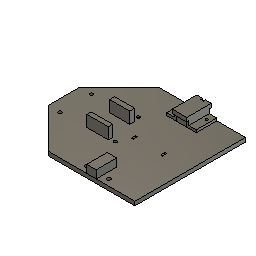
Chassis_v1 v17 (Autodesk Fusion 360 design; units mm, degrees)
Autodesk Fusion 360 part; units mm, degrees
sketch "Sketch1" plane through (0, 0, 0) normal (0, 1, 0) x (1, 0, 0) in component "Chassis"
  line L0 (0, 0) -> (160, 0)
  line L1 (160, 0) -> (160, -140)
  line L2 (160, -140) -> (0, -140)
  line L3 (0, -140) -> (0, 0)
  dimension "d1" = 160
  dimension "d2" = 140
  constraint horizontal L0
  constraint vertical L1
  constraint horizontal L2
  constraint vertical L3
  constraint coincident L0.start L3.end
  measures "d1" distance of L0.start L0.end
  measures "d2" distance of L0.start L2.end
extrude "Extrude1" add sketch "Sketch1" along normal blind 5.08 makes body 1 in component "Chassis"
sketch "Sketch2" plane through (0, 5.08, 0) normal (0, 1, 0) x (-1, 0, 0) in component "Chassis"
  line L0 (0, 140) -> (-160, 140)
  line L1 (-160, 140) -> (-160, 0)
  line L2 (-160, 0) -> (0, 0)
  line L3 (0, 0) -> (0, 140)
  line L4 (-80, 0) -> (-80, 140) construction
  line L5 (0, 70) -> (-160, 70) construction
  line L6 (-160, 0) -> (0, 140) construction
  line L7 (0, 0) -> (-160, 140) construction
  circle A0 centre (-15, 50.275) radius 2
  circle A1 centre (-15, 89.725) radius 2
  line L8 (-15, 50.275) -> (-15, 89.725) construction
  line L9 (-15, 70) -> (-20, 70) construction
  dimension "d5" = 4
  dimension "d6" = 4
  dimension "d7" = 39.45
  dimension "d8" = 15
  dimension "d9" = 15
  constraint midpoint L2 L4.start
  constraint midpoint L0 L4.end
  constraint midpoint L3 L5.start
  constraint midpoint L1 L5.end
  constraint coincident L1.end L2.start
  constraint coincident L0.start L3.end
  constraint coincident L2.end L3.start
  constraint coincident L0.end L1.start
  constraint coincident A0.centre L8.start
  constraint coincident A1.centre L8.end
  constraint midpoint L8 L9.start
  constraint perpendicular L8 L9
  constraint collinear L5 L9
  measures "d5" diameter of A0
  measures "d6" diameter of A1
  measures "d7" vertical distance of A0.centre A1.centre
  measures "d8" distance of L3 A0.centre
  measures "d9" distance of L3 A1.centre
extrude "Extrude2" cut sketch "Sketch2" against normal blind 5.08 contours A0 | A1 bodies 1 in component "Chassis"
sketch "Sketch3" plane through (0, 5.08, 0) normal (0, 1, 0) x (-1, 0, 0) in component "Chassis"
  circle A0 centre (-15, 50.275) radius 2
  circle A1 centre (-15, 89.725) radius 2
  line L0 (0, 140) -> (-160, 140)
  line L1 (-160, 140) -> (-160, 0)
  line L2 (-160, 0) -> (0, 0)
  line L3 (0, 0) -> (0, 140)
  line L4 (-30, 71.55) -> (-84, 71.55) construction
  line L5 (-84, 71.55) -> (-84, 109.55) construction
  line L6 (-84, 109.55) -> (-30, 109.55) construction
  line L7 (-30, 109.55) -> (-30, 71.55) construction
  circle A2 centre (-82.2, 86.84) radius 2
  circle A3 centre (-42.6, 80.03) radius 2
  line L8 (0, 70) -> (-160, 70) construction
  dimension "d12" = 54
  dimension "d13" = 38
  dimension "d14" = 4
  dimension "d15" = 22.71
  dimension "d16" = 1.8
  dimension "d17" = 4
  dimension "d18" = 8.48
  dimension "d19" = 12.6
  dimension "d20" = 30.45
  dimension "d21" = 30
  constraint horizontal L4
  constraint vertical L5
  constraint horizontal L6
  constraint vertical L7
  constraint midpoint L3 L8.start
  constraint midpoint L1 L8.end
  measures "d12" distance of L5.end L6.end
  measures "d13" distance of L4.start L6.end
  measures "d14" diameter of A2
  measures "d15" distance of L6 A2.centre
  measures "d16" distance of L5 A2.centre
  measures "d17" diameter of A3
  measures "d18" distance of L4 A3.centre
  measures "d19" distance of L7 A3.centre
  measures "d20" distance of L0 L6
  measures "d21" distance of L3 L7
extrude "Extrude3" cut sketch "Sketch3" against normal blind 5.08 contours A2 | A3 bodies 1 in component "Chassis"
sketch "Sketch4" plane through (0, 0, 0) normal (0, -1, 0) x (1, 0, 0) in component "Chassis"
  circle A0 centre (42.6, 80.03) radius 2
  circle A1 centre (82.2, 86.84) radius 2
  circle A2 centre (15, 50.275) radius 2
  circle A3 centre (15, 89.725) radius 2
  line L0 (160, 140) -> (0, 140)
  line L1 (0, 140) -> (0, 0)
  line L2 (0, 0) -> (160, 0)
  line L3 (160, 0) -> (160, 140)
  circle A4 centre (42.6, 80.03) radius 5
  circle A5 centre (82.2, 86.84) radius 5
  point P0 (42.6, 80.03)
  point P1 (82.2, 86.84)
  dimension "d105" = 10
  dimension "d106" = 10
  constraint coincident P0 A0.centre
  constraint coincident P1 A1.centre
  constraint concentric A1 A5
  measures "d105" diameter of A4
  measures "d106" diameter of A5
extrude "Extrude10" cut sketch "Sketch4" against normal blind 3 contours A4 | A5 bodies 1 in component "Chassis"
extrude "Extrude4" cut sketch "Sketch4" against normal blind 3 contours A0 | A4 | A5 bodies 1 in component "Chassis"
chamfer "Chamfer1" distance 50 angle 45 2 edges at (0, 2.54, 140) (0, 2.54, 0) on bodies 1 in component "Chassis"
sketch "Sketch5" plane through (0, 5.08, 0) normal (0, 1, 0) x (-1, 0, 0) in component "Chassis"
  line L0 (-93, 41.4) -> (-123, 41.4) construction
  line L1 (-123, 41.4) -> (-123, 98.6) construction
  line L2 (-123, 98.6) -> (-93, 98.6) construction
  line L3 (-93, 98.6) -> (-93, 41.4) construction
  line L4 (-123, 70) -> (-93, 70) construction
  line L5 (0, 70) -> (-160, 70) construction
  line L6 (-84, 71.55) -> (-84, 109.55)
  line L7 (-91, 72.5) -> (-88.5, 72.5)
  line L8 (-88.5, 72.5) -> (-88.5, 67.5)
  line L9 (-88.5, 67.5) -> (-91, 67.5)
  line L10 (-91, 67.5) -> (-91, 72.5)
  line L11 (-91, 72.5) -> (-88.5, 67.5) construction
  line L12 (-88.5, 72.5) -> (-91, 67.5) construction
  line L13 (-128, 72.5) -> (-125.5, 72.5)
  line L14 (-125.5, 72.5) -> (-125.5, 67.5)
  line L15 (-125.5, 67.5) -> (-128, 67.5)
  line L16 (-128, 67.5) -> (-128, 72.5)
  line L17 (-128, 72.5) -> (-125.5, 67.5) construction
  line L18 (-125.5, 72.5) -> (-128, 67.5) construction
  point P0 (-89.75, 70)
  point P1 (-126.75, 70)
  dimension "d29" = 30
  dimension "d30" = 57.2
  dimension "d31" = 9
  dimension "d32" = 2.5
  dimension "d33" = 5
  dimension "d34" = 2
  dimension "d35" = 2.5
  dimension "d36" = 5
  dimension "d37" = 2.5
  constraint horizontal L0
  constraint vertical L1
  constraint horizontal L2
  constraint vertical L3
  constraint midpoint L1 L4.start
  constraint midpoint L3 L4.end
  constraint collinear L4 L5
  constraint horizontal L7
  constraint perpendicular L7 L8
  constraint parallel L7 L9
  constraint parallel L8 L10
  constraint coincident L11 P0
  constraint coincident L12 P0
  constraint coincident L5 P0
  constraint horizontal L13
  constraint perpendicular L13 L14
  constraint parallel L13 L15
  constraint parallel L14 L16
  constraint coincident L17 P1
  constraint coincident L18 P1
  constraint coincident L5 P1
  measures "d29" distance of L0.start L0.end
  measures "d30" distance of L0.start L2.end
  measures "d31" distance of L3 L6
  measures "d32" distance of L8.end L9.end
  measures "d33" distance of L7.end L8.end
  measures "d34" distance of L3 L10
  measures "d35" distance of L14.end L15.end
  measures "d36" distance of L13.end L14.end
  measures "d37" distance of L1 L14
extrude "Extrude5" cut sketch "Sketch5" against normal blind 5.08 bodies 1 in component "Chassis"
sketch "Sketch6" plane through (0, 5.08, 0) normal (0, 1, 0) x (-1, 0, 0) in component "Chassis"
  line L0 (-47, 43.05) -> (-72.4, 43.05) construction
  line L1 (-72.4, 43.05) -> (-72.4, 68.45) construction
  line L2 (-72.4, 68.45) -> (-47, 68.45) construction
  line L3 (-47, 68.45) -> (-47, 43.05) construction
  line L4 (0, 70) -> (-160, 70)
  line L5 (0, 0) -> (0, 140)
  circle A0 centre (-49.54, 45.59) radius 2
  circle A1 centre (-69.86, 45.59) radius 2
  line L6 (-59.7, 43.05) -> (-59.7, 68.45) construction
  line L7 (-47, 55.75) -> (-72.4, 55.75) construction
  line L8 (-72.4, 58.925) -> (-47, 58.925)
  line L9 (-47, 58.925) -> (-47, 52.575)
  line L10 (-47, 52.575) -> (-72.4, 52.575)
  line L11 (-72.4, 52.575) -> (-72.4, 58.925)
  line L12 (-72.4, 58.925) -> (-47, 52.575) construction
  line L13 (-47, 58.925) -> (-72.4, 52.575) construction
  point P0 (-59.7, 55.75)
  dimension "d40" = 25.4
  dimension "d41" = 25.4
  dimension "d42" = 1.55
  dimension "d43" = 47
  dimension "d44" = 4
  dimension "d45" = 2.54
  dimension "d46" = 2.54
  dimension "d47" = 4
  dimension "d48" = 2.54
  dimension "d49" = 2.54
  dimension "d52" = 6.35
  constraint horizontal L0
  constraint vertical L1
  constraint horizontal L2
  constraint vertical L3
  constraint midpoint L0 L6.start
  constraint midpoint L2 L6.end
  constraint midpoint L3 L7.start
  constraint midpoint L1 L7.end
  constraint horizontal L8
  constraint perpendicular L8 L9
  constraint parallel L8 L10
  constraint parallel L9 L11
  constraint coincident L12 P0
  constraint coincident L13 P0
  constraint midpoint L7 P0
  measures "d40" distance of L0.start L0.end
  measures "d41" distance of L0.start L2.end
  measures "d42" distance of L2 L4
  measures "d43" distance of L3 L5
  measures "d44" diameter of A0
  measures "d45" distance of L0 A0.centre
  measures "d46" distance of L3 A0.centre
  measures "d47" diameter of A1
  measures "d48" distance of L0 A1.centre
  measures "d49" distance of L1 A1.centre
  measures "d52" distance of L8.end L9.end
extrude "Extrude7" add sketch "Sketch6" along normal blind 14.45 contours L8 L9 L10 L11 bodies 1 in component "Chassis"
extrude "Extrude6" cut sketch "Sketch6" against normal blind 5.08 contours A0 | A1 bodies 1 in component "Chassis"
sketch "Sketch7" plane through (0, 0, 0) normal (0, -1, 0) x (1, 0, 0) in component "Chassis"
  circle A0 centre (49.54, 45.59) radius 2
  circle A1 centre (69.86, 45.59) radius 2
  line L0 (88.5, 67.5) -> (88.5, 72.5)
  line L1 (88.5, 72.5) -> (91, 72.5)
  line L2 (91, 72.5) -> (91, 67.5)
  line L3 (91, 67.5) -> (88.5, 67.5)
  line L4 (125.5, 67.5) -> (125.5, 72.5)
  line L5 (125.5, 72.5) -> (128, 72.5)
  line L6 (128, 72.5) -> (128, 67.5)
  line L7 (128, 67.5) -> (125.5, 67.5)
  line L8 (0, 50) -> (50, 0)
  line L9 (50, 0) -> (160, 0)
  line L10 (160, 0) -> (160, 140)
  line L11 (160, 140) -> (50, 140)
  line L12 (50, 140) -> (0, 90)
  line L13 (0, 90) -> (0, 50)
  circle A2 centre (15, 50.275) radius 2
  circle A3 centre (15, 89.725) radius 2
  circle A4 centre (42.6, 80.03) radius 5
  circle A5 centre (82.2, 86.84) radius 5
  circle A6 centre (49.54, 45.59) radius 5
  circle A7 centre (69.86, 45.59) radius 5
  point P0 (49.54, 45.59)
  point P1 (69.86, 45.59)
  dimension "d109" = 10
  dimension "d110" = 10
  constraint coincident P0 A0.centre
  constraint coincident P1 A1.centre
  constraint concentric A0 A6
  measures "d109" diameter of A6
  measures "d110" diameter of A7
extrude "Extrude11" cut sketch "Sketch7" against normal blind 3 contours A6 | A7 bodies 1 in component "Chassis"
extrude "Extrude8" cut sketch "Sketch7" against normal blind 3 contours A0 | A6 | A7 bodies 1 in component "Chassis"
sketch "Sketch1 (2)" plane through (0, 5.08, 0) normal (0, 1, 0) x (-1, 0, 0) in component "Motor_Right"
  circle A0 centre (-49.54, 45.59) radius 2
  circle A1 centre (-69.86, 45.59) radius 2
  line L0 (-72.4, 52.575) -> (-72.4, 58.925)
  line L1 (-72.4, 58.925) -> (-47, 58.925)
  line L2 (-47, 58.925) -> (-47, 52.575)
  line L3 (-47, 52.575) -> (-72.4, 52.575)
  line L4 (-88.5, 72.5) -> (-88.5, 67.5)
  line L5 (-88.5, 67.5) -> (-91, 67.5)
  line L6 (-91, 67.5) -> (-91, 72.5)
  line L7 (-91, 72.5) -> (-88.5, 72.5)
  line L8 (-125.5, 72.5) -> (-125.5, 67.5)
  line L9 (-125.5, 67.5) -> (-128, 67.5)
  line L10 (-128, 67.5) -> (-128, 72.5)
  line L11 (-128, 72.5) -> (-125.5, 72.5)
  circle A2 centre (-42.6, 80.03) radius 2
  circle A3 centre (-82.2, 86.84) radius 2
  circle A4 centre (-15, 50.275) radius 2
  circle A5 centre (-15, 89.725) radius 2
  line L12 (-50, 0) -> (0, 50)
  line L13 (0, 50) -> (0, 90)
  line L14 (0, 90) -> (-50, 140)
  line L15 (-50, 140) -> (-160, 140)
  line L16 (-160, 140) -> (-160, 0)
  line L17 (-160, 0) -> (-50, 0)
  line L18 (-105, 140) -> (-105, 70) construction
  line L19 (-105, 140) -> (-99, 140) construction
  line L20 (-99, 140) -> (-111, 140)
  line L21 (-111, 140) -> (-111, 114)
  line L22 (-111, 114) -> (-99, 114)
  line L23 (-99, 114) -> (-99, 140)
  dimension "d59" = 26
  dimension "d60" = 12
  dimension "d61" = 49
  constraint midpoint L15 L18.start
  constraint perpendicular L9 L18
  constraint coincident L15 L19.end
  constraint perpendicular L18 L19
  constraint horizontal L20
  constraint vertical L21
  constraint horizontal L22
  constraint vertical L23
  measures "d59" distance of L19.end L22.end
  measures "d60" distance of L19.end L20.end
  measures "d61" distance of L16 L21
extrude "Extrude1'" add sketch "Sketch1 (2)" along normal blind 10 separate body contours L15 L20 L21 L22 L23 makes body 2 in component "Motor_Right"
sketch "Sketch1 (3)" plane through (0, 5.08, 0) normal (0, 1, 0) x (-1, 0, 0) in component "Motor_Left"
  circle A0 centre (-49.54, 45.59) radius 2
  circle A1 centre (-69.86, 45.59) radius 2
  line L0 (-72.4, 52.575) -> (-72.4, 58.925)
  line L1 (-72.4, 58.925) -> (-47, 58.925)
  line L2 (-47, 58.925) -> (-47, 52.575)
  line L3 (-47, 52.575) -> (-72.4, 52.575)
  line L4 (-88.5, 72.5) -> (-88.5, 67.5)
  line L5 (-88.5, 67.5) -> (-91, 67.5)
  line L6 (-91, 67.5) -> (-91, 72.5)
  line L7 (-91, 72.5) -> (-88.5, 72.5)
  line L8 (-125.5, 72.5) -> (-125.5, 67.5)
  line L9 (-125.5, 67.5) -> (-128, 67.5)
  line L10 (-128, 67.5) -> (-128, 72.5)
  line L11 (-128, 72.5) -> (-125.5, 72.5)
  circle A2 centre (-42.6, 80.03) radius 2
  circle A3 centre (-82.2, 86.84) radius 2
  circle A4 centre (-15, 50.275) radius 2
  circle A5 centre (-15, 89.725) radius 2
  line L12 (-50, 0) -> (0, 50)
  line L13 (0, 50) -> (0, 90)
  line L14 (0, 90) -> (-50, 140)
  line L15 (-50, 140) -> (-160, 140)
  line L16 (-160, 140) -> (-160, 0)
  line L17 (-160, 0) -> (-50, 0)
  line L18 (-105, 0) -> (-105, 70) construction
  line L19 (-105, 0) -> (-99, 0) construction
  line L20 (-99, 0) -> (-111, 0)
  line L21 (-111, 0) -> (-111, 26)
  line L22 (-111, 26) -> (-99, 26)
  line L23 (-99, 26) -> (-99, 0)
  dimension "d64" = 6
  dimension "d65" = 12
  dimension "d66" = 26
  constraint midpoint L17 L18.start
  constraint perpendicular L17 L18
  constraint perpendicular L18 L19
  constraint horizontal L20
  constraint vertical L21
  constraint horizontal L22
  constraint vertical L23
  measures "d64" distance of L18.start L19.end
  measures "d65" distance of L19.end L20.end
  measures "d66" distance of L19.end L22.end
extrude "Extrude1''" add sketch "Sketch1 (3)" along normal blind 10 separate body contours L17 L20 L21 L22 L23 makes body 3 in component "Motor_Left"
sketch "Sketch1 (4)" plane through (0, 0, 0) normal (0, 0, -1) x (-1, 0, 0) in component "Motor_Bracket_Left"
  line L0 (-111, 5.08) -> (-99, 5.08)
  line L1 (-99, 5.08) -> (-99, 15.08)
  line L2 (-99, 15.08) -> (-111, 15.08)
  line L3 (-111, 15.08) -> (-111, 5.08)
  line L4 (-111.03, 15.11) -> (-111.03, 5.08)
  line L5 (-160, 5.08) -> (-50, 5.08)
  line L6 (-111.03, 5.08) -> (-123.73, 5.08)
  line L7 (-123.73, 5.08) -> (-123.73, 8.255)
  line L8 (-123.73, 8.255) -> (-114.205, 8.255)
  line L9 (-114.205, 8.255) -> (-114.205, 18.285)
  line L10 (-105, 18.285) -> (-114.205, 18.285)
  line L11 (-105, 15.11) -> (-111.03, 15.11)
  line L12 (-105, 18.285) -> (-95.795, 18.285)
  line L13 (-95.795, 8.255) -> (-95.795, 18.285)
  line L14 (-86.27, 8.255) -> (-95.795, 8.255)
  line L15 (-86.27, 5.08) -> (-86.27, 8.255)
  line L16 (-105, 15.11) -> (-98.97, 15.11)
  line L17 (-98.97, 15.11) -> (-98.97, 5.08)
  line L18 (-98.97, 5.08) -> (-86.27, 5.08)
  dimension "d70" = 12.7
  dimension "d71" = 3.175
  dimension "d72" = 9.525
  dimension "d73" = 10.03
  dimension "d74" = 10.03
  dimension "d75" = 18.41
  dimension "d76" = 37.46
  dimension "d77" = 13.205
  constraint parallel L3 L4
  constraint coincident L4.end L5
  constraint perpendicular L4 L6
  constraint perpendicular L5 L7
  constraint perpendicular L7 L8
  constraint perpendicular L8 L9
  constraint perpendicular L9 L10
  measures "d70" distance of L4.end L6.end
  measures "d71" distance of L6.end L7.end
  measures "d72" distance of L7.end L8.end
  measures "d73" distance of L4.end L4.start
  measures "d74" distance of L8.end L9.end
  measures "d75" distance of L9 L13
  measures "d76" distance of L7 L15
  measures "d77" distance of L12 L18
extrude "Extrude1'''" add sketch "Sketch1 (4)" against normal blind 16 separate body contours L4 L5 L6 L7 L8 L9 L10 L11 L12 L13 L14 L15 L16 L17 L18 makes body 4 in component "Motor_Bracket_Left"
sketch "Sketch2 (2)" plane through (0, 0, 0) normal (0, 0, -1) x (-1, 0, 0) in component "Motor_Bracket_Left"
  line L0 (-111.03, 15.11) -> (-98.97, 15.11)
  line L1 (-98.97, 15.11) -> (-98.97, 5.08)
  line L2 (-98.97, 5.08) -> (-86.27, 5.08)
  line L3 (-86.27, 5.08) -> (-86.27, 8.255)
  line L4 (-86.27, 8.255) -> (-95.795, 8.255)
  line L5 (-95.795, 8.255) -> (-95.795, 18.285)
  line L6 (-95.795, 18.285) -> (-114.205, 18.285)
  line L7 (-114.205, 18.285) -> (-114.205, 8.255)
  line L8 (-114.205, 8.255) -> (-123.73, 8.255)
  line L9 (-123.73, 8.255) -> (-123.73, 5.08)
  line L10 (-123.73, 5.08) -> (-111.03, 5.08)
  line L11 (-111.03, 5.08) -> (-111.03, 15.11)
  line L12 (-114.205, 18.285) -> (-95.795, 18.285)
  line L13 (-95.795, 18.285) -> (-95.795, 13.27)
  line L14 (-95.795, 13.27) -> (-114.205, 13.27)
  line L15 (-114.205, 13.27) -> (-114.205, 18.285)
  dimension "d121" = 5.015
  dimension "d122" = 18.41
  constraint horizontal L12
  constraint vertical L13
  constraint horizontal L14
  constraint vertical L15
  constraint midpoint L5 L13.end
  constraint coincident L6.end L7.start
  measures "d121" distance of L6.end L14.end
  measures "d122" distance of L6.end L5.end
extrude "Extrude2'" add sketch "Sketch2 (2)" along normal blind 2.5 contours L0 L1 L5 L6 L7 L11 L12 L13 L14 L15 | L0 L1 L11 L14 bodies 4 in component "Motor_Bracket_Left"
sketch "Sketch3 (2)" plane through (0, 13.27, 0) normal (0, -1, 0) x (1, 0, 0) in component "Motor_Bracket_Left"
  line L0 (98.97, 0) -> (95.795, 0)
  line L1 (95.795, 0) -> (95.795, -2.5)
  line L2 (95.795, -2.5) -> (114.205, -2.5)
  line L3 (114.205, -2.5) -> (114.205, 0)
  line L4 (114.205, 0) -> (111.03, 0)
  line L5 (111.03, 0) -> (98.97, 0)
  line L6 (105, -2.5) -> (105, 0) construction
  line L7 (95.795, -1.25) -> (114.205, -1.25) construction
  line L8 (109.875, -2.5) -> (100.125, -2.5)
  line L9 (100.125, -2.5) -> (100.125, 0)
  line L10 (100.125, 0) -> (109.875, 0)
  line L11 (109.875, 0) -> (109.875, -2.5)
  line L12 (109.875, -2.5) -> (100.125, 0) construction
  line L13 (100.125, -2.5) -> (109.875, 0) construction
  point P0 (105, -1.25)
  dimension "d82" = 9.75
  constraint midpoint L2 L6.start
  constraint midpoint L5 L6.end
  constraint midpoint L1 L7.start
  constraint midpoint L3 L7.end
  constraint horizontal L8
  constraint perpendicular L8 L9
  constraint parallel L8 L10
  constraint parallel L9 L11
  constraint coincident L12 P0
  constraint coincident L13 P0
  constraint midpoint L7 P0
  measures "d82" distance of L9.end L10.end
extrude "Extrude3'" cut sketch "Sketch3 (2)" against normal blind 1.84 contours L2 L5 L8 L9 L10 L11 bodies 4 in component "Motor_Bracket_Left"
sketch "Sketch4 (2)" plane through (0, 8.255, 0) normal (0, 1, 0) x (-1, 0, 0) in component "Motor_Bracket_Left"
  line L0 (-123.73, 0) -> (-114.205, 0)
  line L1 (-114.205, 0) -> (-114.205, 16)
  line L2 (-114.205, 16) -> (-123.73, 16)
  line L3 (-123.73, 16) -> (-123.73, 0)
  line L4 (-114.205, 0) -> (-123.73, 16) construction
  line L5 (-123.73, 0) -> (-114.205, 16) construction
  circle A0 centre (-118.9675, 8) radius 1.5
  dimension "d85" = 3
  constraint coincident L0.end L1.start
  constraint coincident L2.end L3.start
  constraint coincident L0.start L3.end
  constraint coincident L1.end L2.start
  constraint midpoint L5 A0.centre
  measures "d85" diameter of A0
extrude "Extrude4'" cut sketch "Sketch4 (2)" against normal blind 3.175 contours A0 bodies 4 in component "Motor_Bracket_Left"
sketch "Sketch5 (2)" plane through (0, 8.255, 0) normal (0, 1, 0) x (-1, 0, 0) in component "Motor_Bracket_Left"
  line L0 (-95.795, 0) -> (-86.27, 0)
  line L1 (-86.27, 0) -> (-86.27, 16)
  line L2 (-86.27, 16) -> (-95.795, 16)
  line L3 (-95.795, 16) -> (-95.795, 0)
  line L4 (-86.27, 16) -> (-95.795, 0) construction
  line L5 (-86.27, 0) -> (-95.795, 16) construction
  circle A0 centre (-91.0325, 8) radius 1.5
  dimension "d88" = 3
  constraint coincident L1.end L2.start
  constraint coincident L0.start L3.end
  constraint coincident L0.end L1.start
  constraint coincident L2.end L3.start
  constraint midpoint L4 A0.centre
  measures "d88" diameter of A0
extrude "Extrude5'" cut sketch "Sketch5 (2)" against normal blind 3.175 contours A0 bodies 4 in component "Motor_Bracket_Left"
extrude "Extrude6'" add 1 faces at (107.01, 17.2267, 16) along direction (0, 0, 1) blind 10.03 on bodies 4 bodies 4 in component "Motor_Bracket_Left"
sketch "Sketch6 (2)" plane through (0, 0, 26.03) normal (0, 0, 1) x (1, 0, 0) in component "Motor_Bracket_Left"
  line L0 (98.97, 15.11) -> (111.03, 15.11)
  line L1 (111.03, 15.11) -> (111.03, 5.08)
  line L2 (111.03, 5.08) -> (123.73, 5.08)
  line L3 (123.73, 5.08) -> (123.73, 8.255)
  line L4 (123.73, 8.255) -> (114.205, 8.255)
  line L5 (114.205, 8.255) -> (114.205, 18.285)
  line L6 (114.205, 18.285) -> (95.795, 18.285)
  line L7 (95.795, 18.285) -> (95.795, 8.255)
  line L8 (95.795, 8.255) -> (86.27, 8.255)
  line L9 (86.27, 8.255) -> (86.27, 5.08)
  line L10 (86.27, 5.08) -> (98.97, 5.08)
  line L11 (98.97, 5.08) -> (98.97, 15.11)
  line L12 (95.795, 18.285) -> (114.205, 18.285)
  line L13 (114.205, 18.285) -> (114.205, 13.27)
  line L14 (114.205, 13.27) -> (95.795, 13.27)
  line L15 (95.795, 13.27) -> (95.795, 18.285)
  dimension "d123" = 18.41
  dimension "d124" = 5.015
  constraint horizontal L12
  constraint vertical L13
  constraint horizontal L14
  constraint vertical L15
  constraint midpoint L5 L13.end
  constraint coincident L6.end L7.start
  measures "d123" distance of L6.end L5.end
  measures "d124" distance of L5.end L13.end
extrude "Extrude7'" add sketch "Sketch6 (2)" along normal blind 2.5 contours L0 L1 L5 L6 L7 L11 L12 L13 L14 L15 | L0 L1 L11 L14 bodies 4 in component "Motor_Bracket_Left"
extrude "Extrude8'" cut 2 faces at (99.74, 14.4967, 0) (110.645, 14.4967, 0) along direction (0, 0, -1) blind 0.03 on bodies 4 bodies 4 in component "Motor_Bracket_Left"
sketch "Sketch8" plane through (0, 0, 0) normal (0, -1, 0) x (1, 0, 0) in component "Chassis"
  line L0 (88.5, 67.5) -> (88.5, 72.5)
  line L1 (88.5, 72.5) -> (91, 72.5)
  line L2 (91, 72.5) -> (91, 67.5)
  line L3 (91, 67.5) -> (88.5, 67.5)
  line L4 (125.5, 67.5) -> (125.5, 72.5)
  line L5 (125.5, 72.5) -> (128, 72.5)
  line L6 (128, 72.5) -> (128, 67.5)
  line L7 (128, 67.5) -> (125.5, 67.5)
  line L8 (0, 50) -> (50, 0)
  line L9 (50, 0) -> (160, 0)
  line L10 (160, 0) -> (160, 140)
  line L11 (160, 140) -> (50, 140)
  line L12 (50, 140) -> (0, 90)
  line L13 (0, 90) -> (0, 50)
  circle A0 centre (15, 50.275) radius 2
  circle A1 centre (15, 89.725) radius 2
  circle A2 centre (118.9675, 8) radius 1.5 construction
  circle A3 centre (91.0325, 8) radius 1.5 construction
  circle A4 centre (118.9675, 8) radius 2.15
  circle A5 centre (91.0325, 8) radius 2.15
  line L14 (0, 70) -> (160, 70) construction
  circle A6 centre (118.9675, 132) radius 2.15
  circle A7 centre (91.0325, 132) radius 2.15
  circle A8 centre (91.0325, 132) radius 2.15
  circle A9 centre (118.9675, 132) radius 2.15
  circle A10 centre (91.0325, 8) radius 2.15
  circle A11 centre (118.9675, 8) radius 2.15
  circle A12 centre (42.6, 80.03) radius 5
  circle A13 centre (82.2, 86.84) radius 5
  circle A14 centre (69.86, 45.59) radius 5
  circle A15 centre (49.54, 45.59) radius 5
  dimension "d97" = 4.3
  dimension "d98" = 4.3
  constraint concentric A2 A4
  constraint concentric A3 A5
  constraint midpoint L13 L14.start
  constraint midpoint L10 L14.end
  constraint symmetric A4 L14 A6
  constraint symmetric A5 L14 A7
  constraint concentric A7 A8
  constraint concentric A6 A9
  constraint concentric A5 A10
  constraint concentric A2 A11
  measures "d97" diameter of A4
  measures "d98" diameter of A5
sketch "Sketch9" plane through (0, 5.08, 0) normal (0, 1, 0) x (-1, 0, 0) in component "Chassis"
  circle A0 centre (-49.54, 45.59) radius 2
  circle A1 centre (-69.86, 45.59) radius 2
  line L0 (-72.4, 52.575) -> (-72.4, 58.925)
  line L1 (-72.4, 58.925) -> (-47, 58.925)
  line L2 (-47, 58.925) -> (-47, 52.575)
  line L3 (-47, 52.575) -> (-72.4, 52.575)
  line L4 (-88.5, 72.5) -> (-88.5, 67.5)
  line L5 (-88.5, 67.5) -> (-91, 67.5)
  line L6 (-91, 67.5) -> (-91, 72.5)
  line L7 (-91, 72.5) -> (-88.5, 72.5)
  line L8 (-125.5, 72.5) -> (-125.5, 67.5)
  line L9 (-125.5, 67.5) -> (-128, 67.5)
  line L10 (-128, 67.5) -> (-128, 72.5)
  line L11 (-128, 72.5) -> (-125.5, 72.5)
  circle A2 centre (-42.6, 80.03) radius 2
  circle A3 centre (-82.2, 86.84) radius 2
  circle A4 centre (-15, 50.275) radius 2
  circle A5 centre (-15, 89.725) radius 2
  line L12 (-50, 0) -> (0, 50)
  line L13 (0, 50) -> (0, 90)
  line L14 (0, 90) -> (-50, 140)
  line L15 (-50, 140) -> (-160, 140)
  line L16 (-160, 140) -> (-160, 0)
  line L17 (-160, 0) -> (-50, 0)
  circle A6 centre (-91, 8) radius 2.15
  circle A7 centre (-119, 8) radius 2.15
  circle A8 centre (-91, 132) radius 2.15
  circle A9 centre (-119, 132) radius 2.15
  dimension "d99" = 4.3
  dimension "d100" = 4.3
  dimension "d101" = 4.3
  dimension "d102" = 4.3
  measures "d99" diameter of A6
  measures "d100" diameter of A7
  measures "d101" diameter of A8
  measures "d102" diameter of A9
extrude "Extrude9" cut sketch "Sketch9" against normal blind 3.43 contours A6 | A7 | A8 | A9 bodies 1 in component "Chassis"
sketch "Sketch7 (2)" plane through (0, 0, -2.5) normal (0, 0, -1) x (-1, 0, 0) in component "Motor_Bracket_Left"
  line L0 (-109.875, 13.27) -> (-109.875, 15.11)
  line L1 (-109.875, 15.11) -> (-100.125, 15.11)
  line L2 (-100.125, 15.11) -> (-100.125, 13.27)
  line L3 (-100.125, 13.27) -> (-95.795, 13.27)
  line L4 (-95.795, 13.27) -> (-95.795, 18.285)
  line L5 (-95.795, 18.285) -> (-114.205, 18.285)
  line L6 (-114.205, 18.285) -> (-114.205, 13.27)
  line L7 (-114.205, 13.27) -> (-109.875, 13.27)
  line L8 (-105, 15.11) -> (-105, 18.285) construction
  line L9 (-105, 16.6975) -> (-114.205, 16.6975) construction
  line L10 (-103.5, 15.11) -> (-106.5, 15.11)
  line L11 (-106.5, 15.11) -> (-106.5, 18.285)
  line L12 (-106.5, 18.285) -> (-103.5, 18.285)
  line L13 (-103.5, 18.285) -> (-103.5, 15.11)
  line L14 (-103.5, 15.11) -> (-106.5, 18.285) construction
  line L15 (-106.5, 15.11) -> (-103.5, 18.285) construction
  point P0 (-105, 16.6975)
  dimension "d113" = 3
  constraint midpoint L1 L8.start
  constraint midpoint L5 L8.end
  constraint midpoint L8 P0
  constraint coincident L6 L9.end
  constraint perpendicular L6 L9
  constraint horizontal L10
  constraint perpendicular L10 L11
  constraint parallel L10 L12
  constraint parallel L11 L13
  constraint coincident L14 P0
  constraint coincident L15 P0
  constraint coincident P0 L9.start
  measures "d113" distance of L11.end L12.end
extrude "Extrude9'" cut sketch "Sketch7 (2)" against normal blind 2.5 contours L1 L5 L10 L11 L12 L13 bodies 4 in component "Motor_Bracket_Left"
sketch "Sketch10" plane through (0, 5.08, 0) normal (0, 1, 0) x (-1, 0, 0) in component "Chassis"
  circle A0 centre (-119, 132) radius 2.15
  circle A1 centre (-91, 8) radius 2.15
  circle A2 centre (-91, 132) radius 2.15
  circle A3 centre (-119, 8) radius 2.15
  circle A4 centre (-49.54, 45.59) radius 2
  circle A5 centre (-69.86, 45.59) radius 2
  line L0 (-72.4, 52.575) -> (-72.4, 58.925)
  line L1 (-72.4, 58.925) -> (-47, 58.925)
  line L2 (-47, 58.925) -> (-47, 52.575)
  line L3 (-47, 52.575) -> (-72.4, 52.575)
  line L4 (-88.5, 72.5) -> (-88.5, 67.5)
  line L5 (-88.5, 67.5) -> (-91, 67.5)
  line L6 (-91, 67.5) -> (-91, 72.5)
  line L7 (-91, 72.5) -> (-88.5, 72.5)
  line L8 (-125.5, 72.5) -> (-125.5, 67.5)
  line L9 (-125.5, 67.5) -> (-128, 67.5)
  line L10 (-128, 67.5) -> (-128, 72.5)
  line L11 (-128, 72.5) -> (-125.5, 72.5)
  circle A6 centre (-42.6, 80.03) radius 2
  circle A7 centre (-82.2, 86.84) radius 2
  circle A8 centre (-15, 50.275) radius 2
  circle A9 centre (-15, 89.725) radius 2
  line L12 (-50, 0) -> (0, 50)
  line L13 (0, 50) -> (0, 90)
  line L14 (0, 90) -> (-50, 140)
  line L15 (-50, 140) -> (-160, 140)
  line L16 (-160, 140) -> (-160, 0)
  line L17 (-160, 0) -> (-50, 0)
  line L18 (-82.2, 86.84) -> (-42.6, 86.84) construction
  line L19 (-62.4, 86.84) -> (-62.4, 83) construction
  line L20 (-48.9, 84.09) -> (-75.9, 84.09)
  line L21 (-75.9, 84.09) -> (-75.9, 89.59)
  line L22 (-75.9, 89.59) -> (-48.9, 89.59)
  line L23 (-48.9, 89.59) -> (-48.9, 84.09)
  line L24 (-48.9, 84.09) -> (-75.9, 89.59) construction
  line L25 (-75.9, 84.09) -> (-48.9, 89.59) construction
  point P0 (-62.4, 86.84)
  dimension "d116" = 27
  dimension "d117" = 5.5
  dimension "d120" = 6.3
  constraint coincident A7.centre L18.start
  constraint horizontal L18
  constraint midpoint L18 P0
  constraint perpendicular L18 L19
  constraint horizontal L20
  constraint perpendicular L20 L21
  constraint parallel L20 L22
  constraint parallel L21 L23
  constraint coincident L24 P0
  constraint coincident L25 P0
  constraint coincident P0 L19.start
  measures "d116" distance of L21.end L22.end
  measures "d117" distance of L20.end L21.end
  measures "d120" distance of A7.centre L21
extrude "Extrude12" add sketch "Sketch10" along normal blind 14.45 contours L20 L21 L22 L23 bodies 1 in component "Chassis"
component "Chassis" placed x (1, 0, 0) y (0, 1, 0) z (0, 0, 1) at (0, 0, 0)
component "Motor_Bracket_Left" placed x (1, 0, 0) y (0, 1, 0) z (0, 0, 1) at (0, 0, 0)
component "Motor_Bracket_Right" placed x (1, 0, 0) y (0, 1, 0) z (0, 0, 1) at (0, 0, 0)
component "Motor_Right" placed x (1, 0, 0) y (0, 1, 0) z (0, 0, 1) at (0, 0, 0)
component "Motor_Left" placed x (1, 0, 0) y (0, 1, 0) z (0, 0, 1) at (0, 0, 0)
